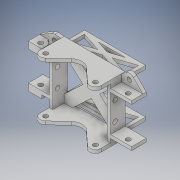
# Autodesk Inventor part: 14HM08 Chassis
Saved by Autodesk Inventor 2019 (Build 230136000, 136)
## iProperties
Created: 2019-01-31
Part Number: 14HM08 Chassis
Material: Generic
Document SubType Name: Modeling
Designer: Billy
Density: 1 g/cm^3
Appearance: Red
Author: Billy
Autodesk Inventor part; units mm, degrees
ref_plane "YZ Plane" through (0, 0, 0) normal (1, 0, 0) x (0, 1, 0)
ref_plane "XZ Plane" through (0, 0, 0) normal (0, 1, 0) x (-1, 0, 0)
ref_plane "XY Plane" through (0, 0, 0) normal (0, 0, 1) x (1, 0, 0)
sketch "Sketch1" plane through (0, 0, 0) normal (0, 1, 0) x (-1, 0, 0)
  circle A0 centre (21.95, 0) radius 2
  circle A1 centre (-21.95, 0) radius 2
  arc A2 (26.95, 0) -> (18.5331, 3.6504) centre (21.95, 0) ccw
  arc A3 (-18.5331, 3.6504) -> (-26.95, 0) centre (-21.95, 0) ccw
  arc A4 (-6.8337, -7.3007) -> (6.8337, -7.3007) centre (0, 0) ccw
  line L0 (6.8337, -7.3007) -> (18.5331, 3.6504)
  line L1 (-6.8337, -7.3007) -> (-18.5331, 3.6504)
  line L2 (-26.95, 0) -> (-26.95, -18.25)
  line L3 (-26.95, -18.25) -> (26.95, -18.25)
  line L4 (26.95, -18.25) -> (26.95, 0)
  constraints: 10 end point, 6 point on circle, 5 centre point, 4 tangent, 3 coincident, 1 parallel, 5 other
extrude "Extrusion1" add sketch "Sketch1" along normal blind 3
ref_plane "Work Plane1" through (0, 48, 0) normal (0, 1, 0) x (1, 0, 0)
sketch "Sketch2" plane through (0, 48, 0) normal (0, 1, 0) x (1, 0, 0)
  circle A0 centre (21.95, 0) radius 2 projected
  circle A1 centre (-21.95, 0) radius 2 projected
  line L0 (-18.5331, -3.6504) -> (-6.8337, 7.3007) projected
  arc A2 (6.8337, 7.3007) -> (-6.8337, 7.3007) centre (0, 0) ccw projected
  line L1 (6.8337, 7.3007) -> (18.5331, -3.6504) projected
  arc A3 (18.5331, -3.6504) -> (26.95, 0) centre (21.95, 0) ccw projected
  line L2 (26.95, 0) -> (26.95, 18.25) projected
  line L3 (26.95, 18.25) -> (-26.95, 18.25) projected
  line L4 (-26.95, 18.25) -> (-26.95, 0) projected
  arc A4 (-26.95, 0) -> (-18.5331, -3.6504) centre (-21.95, 0) ccw projected
extrude "Extrusion2" add sketch "Sketch2" along normal blind 3
sketch "Sketch3" plane through (26.95, 48, -18.25) normal (0, 0, -1) x (-1, 0, 0)
  line L0 (0, 0) -> (53.9, 0) projected
  line L1 (53.9, 0) -> (53.9, 3) projected
  line L2 (0, 3) -> (53.9, 3) projected
  line L3 (0, 0) -> (0, 3) projected
  line L4 (53.9, -48) -> (0, -48) projected
  line L5 (53.9, -48) -> (53.9, -45) projected
  line L6 (0, -45) -> (53.9, -45) projected
  line L7 (0, -48) -> (0, -45) projected
  circle A0 centre (-6.625, -46.63) radius 2
  circle A1 centre (-6.625, 1.63) radius 2
  circle A2 centre (59.415, -43.455) radius 2
  circle A3 centre (59.415, -1.545) radius 2
  arc A4 (58.9874, -48.4367) -> (59.415, -38.455) centre (59.415, -43.455) ccw
  arc A5 (-6.625, -41.63) -> (-3.6882, -50.6767) centre (-6.625, -46.63) ccw
  arc A6 (59.415, -6.545) -> (58.9874, 3.4367) centre (59.415, -1.545) ccw
  arc A7 (-3.6882, 5.6767) -> (-6.625, -3.37) centre (-6.625, 1.63) ccw
  line L8 (53.9, -48) -> (0, -48)
  line L9 (0, 3) -> (53.9, 3)
  line L10 (0, -48) -> (-3.6882, -50.6767)
  line L11 (-6.625, -41.63) -> (0, -41.63)
  line L12 (53.9, -48) -> (58.9874, -48.4367)
  line L13 (59.415, -38.455) -> (53.9, -38.455)
  line L14 (53.9, -45) -> (53.9, -48)
  line L15 (0, -48) -> (0, -45)
  line L16 (59.415, -6.545) -> (53.9, -6.545)
  line L17 (53.9, 3) -> (58.9874, 3.4367)
  line L18 (53.9, 3) -> (53.9, 0)
  line L19 (53.9, -6.545) -> (53.9, -38.455)
  line L20 (0, 3) -> (-3.6882, 5.6767)
  line L21 (-6.625, -3.37) -> (0, -3.37)
  line L22 (0, -41.63) -> (0, -3.37)
  line L23 (0, 0) -> (0, 3)
  point P0 (26.95, -48)
  constraints: 36 end point, 10 parallel, 10 perpendicular, 8 centre point, 8 point on circle, 6 tangent, 4 coincident, 2 horizontal, 2 vertical, 8 other
extrude "Extrusion3" add sketch "Sketch3" along normal blind 3
sketch "Sketch4" plane through (26.95, 0, 0) normal (1, 0, 0) x (0, 0, -1)
  line L0 (18.25, 3) -> (0, 3) projected
  line L1 (7.3007, 48) -> (10, 48) projected
  line L2 (18.25, 3) -> (8.25, 3)
  line L3 (8.25, 3) -> (8.25, 48)
  line L4 (8.25, 48) -> (18.25, 48)
  line L5 (18.25, 48) -> (18.25, 3)
  point P0 (0, 0)
  dimension "d34" = 10
  constraints: 8 end point, 2 parallel, 1 horizontal, 1 perpendicular, 1 point on line
  measures "d34" distance of L3.end L4.end
extrude "Extrusion4" add sketch "Sketch4" against normal blind 3
sketch "Sketch5" plane through (-26.95, 0, 0) normal (-1, 0, 0) x (0, 0, 1)
  line L0 (-8.25, 3) -> (-18.25, 3) projected
  line L1 (-8.25, 3) -> (-8.25, 48) projected
  line L2 (-18.25, 48) -> (-8.25, 48) projected
  line L3 (-18.25, 3) -> (-18.25, 48) projected
  point P0 (0, 0)
extrude "Extrusion5" add sketch "Sketch5" against normal blind 3
sketch "Sketch6" plane through (26.95, 48, -18.25) normal (0, 0, 1) x (1, 0, 0)
  line L0 (-50.9, -6.8604) -> (-50.9, -38.1396)
  line L1 (-10.3025, -45) -> (-43.5975, -45)
  line L2 (-3, -38.1396) -> (-3, -6.8604)
  line L3 (-10.3025, 0) -> (-43.5975, 0)
  line L4 (-50.9, -38.1396) -> (-34.2525, -22.5)
  line L5 (-26.95, -15.6396) -> (-10.3025, 0)
  line L6 (-10.3025, -45) -> (-26.95, -29.3604)
  line L7 (-34.2525, -22.5) -> (-50.9, -6.8604)
  line L8 (-3, -38.1396) -> (-19.6475, -22.5)
  line L9 (-26.95, -15.6396) -> (-43.5975, 0)
  line L10 (-43.5975, -45) -> (-26.95, -29.3604)
  line L11 (-19.6475, -22.5) -> (-3, -6.8604)
  point P0 (-26.95, -48)
  constraints: 24 end point
extrude "Extrusion6" cut sketch "Sketch6" against normal blind 3
sketch "Sketch8" plane through (26.95, 48, -21.25) normal (0, 0, -1) x (-1, 0, 0)
  line L0 (10.3025, -45) -> (26.95, -29.3604)
  line L1 (26.95, -29.3604) -> (43.5975, -45)
  line L2 (43.5975, -45) -> (10.3025, -45)
  line L3 (43.5975, 0) -> (26.95, -15.6396)
  line L4 (26.95, -15.6396) -> (10.3025, 0)
  line L5 (10.3025, 0) -> (43.5975, 0)
  line L6 (3, -6.8604) -> (19.6475, -22.5)
  line L7 (19.6475, -22.5) -> (3, -38.1396)
  line L8 (3, -38.1396) -> (3, -6.8604)
  line L9 (50.9, -38.1396) -> (34.2525, -22.5)
  line L10 (34.2525, -22.5) -> (50.9, -6.8604)
  line L11 (50.9, -6.8604) -> (50.9, -38.1396)
  circle A0 centre (59.415, -1.545) radius 2
  circle A1 centre (59.415, -43.455) radius 2
  circle A2 centre (-6.625, 1.63) radius 2
  circle A3 centre (-6.625, -46.63) radius 2
  line L12 (0, 3) -> (-3.6882, 5.6767)
  arc A4 (-3.6882, 5.6767) -> (-6.625, -3.37) centre (-6.625, 1.63) ccw
  arc A5 (-6.625, -41.63) -> (-3.6882, -50.6767) centre (-6.625, -46.63) ccw
  line L13 (-3.6882, -50.6767) -> (0, -48)
  line L14 (0, -48) -> (53.9, -48)
  line L15 (53.9, -48) -> (58.9874, -48.4367)
  arc A6 (58.9874, -48.4367) -> (59.415, -38.455) centre (59.415, -43.455) ccw
  line L16 (59.415, -38.455) -> (53.9, -38.455)
  line L17 (57.122, -6.545) -> (59.415, -6.545)
  arc A7 (59.415, -6.545) -> (58.9874, 3.4367) centre (59.415, -1.545) ccw
  line L18 (58.9874, 3.4367) -> (53.9, 3)
  line L19 (53.9, 3) -> (0, 3)
  line L20 (53.9, -40.75) -> (0, -40.75)
  line L21 (53.9, -4.25) -> (0, -4.25)
  line L22 (0, -41.63) -> (0, -43.75)
  line L23 (0, -1.25) -> (0, -4.25)
  line L24 (0, -40.75) -> (0, -41.63)
  line L25 (63.6201, -43.75) -> (57.4369, -43.75)
  line L26 (53.9, -43.75) -> (0, -43.75)
  line L27 (63.6201, -1.25) -> (57.4369, -1.25)
  line L28 (53.9, -1.25) -> (0, -1.25)
  line L29 (53.9, -43.75) -> (53.9, -40.75)
  line L30 (53.9, -4.25) -> (53.9, -1.25)
  point P0 (26.95, -48)
  constraints: 62 end point, 8 centre point, 4 point on circle, 1 point on line, 18 other
extrude "Extrusion7" add sketch "Sketch8" along normal blind 18 contours L26 L22 L24 L20 L0 | L0 L20 L1 L26 | L1 L20 L29 L26 | L28 L30 L21 L3 | L3 L21 L4 L28 | L4 L21 L23 L28
sketch "Sketch9" plane through (-12.1236, 43.75, -21.25) normal (0, -1, 0) x (1, 0, 0)
  line L0 (24.2473, 0) -> (39.0736, 0)
  line L1 (24.2473, 0) -> (0, 0)
  line L2 (-14.8264, 0) -> (0, 0)
  line L3 (-14.8264, 0) -> (-14.8264, -18)
  line L4 (39.0736, -18) -> (-14.8264, -18)
  line L5 (39.0736, 0) -> (39.0736, -18)
  line L6 (-11.8264, -15) -> (-11.8264, -3)
  line L7 (0, -3) -> (24.2473, -3)
  line L8 (36.0736, -3) -> (36.0736, -15)
  line L9 (23.7763, -15) -> (0.471, -15)
  line L10 (-8.5123, -18) -> (-14.1928, -19.897)
  line L11 (38.4401, -19.897) -> (32.7596, -18)
  line L12 (12.1236, -11.1086) -> (0.471, -15)
  line L13 (23.7763, -15) -> (12.1236, -11.1086)
  line L14 (5.8096, -9) -> (-11.8264, -14.8896)
  line L15 (-14.8264, -15.8914) -> (-15.4599, -16.103)
  line L16 (5.8096, -9) -> (-11.8264, -3.1104)
  line L17 (-14.8264, -2.1086) -> (-15.4599, -1.897)
  line L18 (38.4401, 1.897) -> (32.7596, 0)
  line L19 (23.7763, -3) -> (12.1236, -6.8914)
  line L20 (-8.5123, 0) -> (-14.1928, 1.897)
  line L21 (12.1236, -6.8914) -> (0.471, -3)
  line L22 (39.7072, -16.103) -> (39.0736, -15.8914)
  line L23 (36.0736, -14.8896) -> (18.4377, -9)
  line L24 (39.7072, -1.897) -> (39.0736, -2.1086)
  line L25 (36.0736, -3.1104) -> (18.4377, -9)
  point P0 (12.1236, 21.25)
  dimension "d62" = 3
  constraints: 52 end point, 14 point on line
  measures "d62" distance between parallel lines of L4 L9
extrude "Extrusion8" cut sketch "Sketch9" along normal blind 180 and the other way blind 9 contours L6 L16 L14 | L7 L19 L21 | L8 L23 L25 | L9 L12 L13
sketch "Sketch13" plane through (26.95, 48, -21.25) normal (0, 0, -1) x (-1, 0, 0)
  line L0 (-6.625, -3.37) -> (0, -3.37)
  line L1 (0, -3.37) -> (-6.625, -3.37)
  line L2 (-11.625, 1.63) -> (-11.625, -6.37)
  line L3 (-11.625, -6.37) -> (0, -6.37)
  line L4 (0, -6.37) -> (0, -3.37)
  line L5 (0, -1.25) -> (11.633, -1.25) projected
  line L6 (11.633, -1.25) -> (10.3025, 0) projected
  line L7 (10.3025, 0) -> (43.5975, 0) projected
  line L8 (43.5975, 0) -> (42.267, -1.25) projected
  line L9 (42.267, -1.25) -> (53.9, -1.25) projected
  line L10 (53.9, -1.25) -> (53.9, -4.25) projected
  line L11 (53.9, -4.25) -> (39.0736, -4.25) projected
  line L12 (39.0736, -4.25) -> (26.95, -15.6396) projected
  line L13 (26.95, -15.6396) -> (14.8264, -4.25) projected
  line L14 (14.8264, -4.25) -> (0, -4.25) projected
  line L15 (0, -4.25) -> (0, -40.75) projected
  line L16 (0, -40.75) -> (14.8264, -40.75) projected
  line L17 (14.8264, -40.75) -> (26.95, -29.3604) projected
  line L18 (26.95, -29.3604) -> (39.0736, -40.75) projected
  line L19 (39.0736, -40.75) -> (53.9, -40.75) projected
  line L20 (53.9, -40.75) -> (53.9, -43.75) projected
  line L21 (53.9, -43.75) -> (42.267, -43.75) projected
  line L22 (42.267, -43.75) -> (43.5975, -45) projected
  line L23 (43.5975, -45) -> (10.3025, -45) projected
  line L24 (10.3025, -45) -> (11.633, -43.75) projected
  line L25 (11.633, -43.75) -> (0, -43.75) projected
  line L26 (0, -43.75) -> (0, -43.3734)
  line L27 (0, -41.63) -> (-6.625, -41.63)
  arc A0 (-6.625, -41.63) -> (-11.625, -46.63) centre (-6.625, -46.63) ccw
  line L28 (-3.6882, -50.6767) -> (0, -48)
  line L29 (0, -48) -> (53.9, -48) projected
  line L30 (53.9, -48) -> (58.9874, -48.4367) projected
  arc A1 (58.9874, -48.4367) -> (59.415, -38.455) centre (59.415, -43.455) ccw projected
  line L31 (59.415, -38.455) -> (53.9, -38.455) projected
  line L32 (53.9, -38.455) -> (53.9, -6.545) projected
  line L33 (53.9, -6.545) -> (59.415, -6.545) projected
  arc A2 (59.415, -6.545) -> (58.9874, 3.4367) centre (59.415, -1.545) ccw projected
  line L34 (58.9874, 3.4367) -> (53.9, 3) projected
  line L35 (53.9, 3) -> (0, 3) projected
  line L36 (0, 3) -> (-3.6882, 5.6767)
  arc A3 (-11.625, 1.63) -> (-6.625, -3.37) centre (-6.625, 1.63) ccw
  line L37 (-6.625, -3.37) -> (0, -3.37)
  line L38 (0, -3.37) -> (0, -1.25)
  line L39 (3, -6.8604) -> (19.6475, -22.5) projected
  line L40 (19.6475, -22.5) -> (3, -38.1396) projected
  line L41 (3, -38.1396) -> (3, -6.8604) projected
  line L42 (50.9, -38.1396) -> (34.2525, -22.5) projected
  line L43 (34.2525, -22.5) -> (50.9, -6.8604) projected
  line L44 (50.9, -6.8604) -> (50.9, -38.1396) projected
  circle A4 centre (59.415, -1.545) radius 2 projected
  circle A5 centre (59.415, -43.455) radius 2 projected
  circle A6 centre (-6.625, 1.63) radius 2
  circle A7 centre (-6.625, -46.63) radius 2
  line L45 (0, -41.63) -> (-6.625, -41.63)
  line L46 (-11.625, -46.63) -> (-11.625, -38.63)
  line L47 (-11.625, -38.63) -> (0, -38.63)
  line L48 (0, -38.63) -> (0, -41.63)
  point P0 (26.95, -48)
  constraints: 30 end point, 12 centre point, 4 point on circle, 1 point on line
extrude "Extrusion11" add sketch "Sketch13" against normal up to surface (3 mm away) contours L0 L4 L3 L2 A3 | L15 L48 L27 A0 L46 L47
sketch "Sketch14" plane through (26.95, 48, -18.25) normal (0, 0, 1) x (1, 0, 0)
  line L0 (0, -48) -> (0, -38.63) projected
  line L1 (3.6882, -50.6767) -> (0, -48) projected
  arc A0 (3.6882, -50.6767) -> (11.625, -46.63) centre (6.625, -46.63) ccw projected
  line L2 (11.625, -38.63) -> (11.625, -46.63) projected
  line L3 (0, -38.63) -> (11.625, -38.63) projected
  circle A1 centre (6.625, -46.63) radius 2 projected
  circle A2 centre (6.625, 1.63) radius 2 projected
  line L4 (0, -6.37) -> (0, 3) projected
  line L5 (11.625, -6.37) -> (0, -6.37) projected
  line L6 (11.625, 1.63) -> (11.625, -6.37) projected
  arc A3 (11.625, 1.63) -> (3.6882, 5.6767) centre (6.625, 1.63) ccw projected
  line L7 (0, 3) -> (3.6882, 5.6767) projected
  line L8 (0, -1.25) -> (0, -4.25) projected
  line L9 (11.625, -6.37) -> (0, -6.37)
  line L10 (0, -6.37) -> (0, -3.37)
  line L11 (0, -3.37) -> (11.625, -3.37)
  line L12 (11.625, -3.37) -> (11.625, -6.37)
  line L13 (11.625, -38.63) -> (0, -38.63)
  line L14 (0, -38.63) -> (0, -41.63)
  line L15 (0, -41.63) -> (11.625, -41.63)
  line L16 (11.625, -41.63) -> (11.625, -38.63)
  point P0 (-26.95, -48)
  dimension "d92" = 3
  dimension "d93" = 3
  constraints: 16 end point, 4 parallel, 2 horizontal, 2 perpendicular, 2 point on line
  measures "d92" distance of L9.end L10.end
  measures "d93" distance of L14.end L13.end
extrude "Extrusion12" add sketch "Sketch14" along normal blind 10 contours L0 L3 L2 L15 | L4 L11 L6 L5
sketch "Sketch15" plane through (38.575, 41.63, -21.25) normal (1, 0, 0) x (0, 0, -1)
  line L0 (-3, -35.26) -> (-3, -40.26) projected
  line L1 (-3, -40.26) -> (0, -40.26) projected
  line L2 (0, -32.26) -> (0, -40.26) projected
  line L3 (0, -32.26) -> (-13, -32.26) projected
  line L4 (-13, -35.26) -> (-13, -32.26) projected
  line L5 (-3, -35.26) -> (-13, -35.26) projected
  line L6 (-3, 8) -> (-3, 3) projected
  line L7 (-3, 3) -> (-13, 3) projected
  line L8 (-13, 0) -> (-13, 3) projected
  line L9 (0, 0) -> (-13, 0) projected
  line L10 (0, 8) -> (0, 0) projected
  line L11 (-3, 8) -> (0, 8) projected
  line L12 (0, -32.26) -> (-13, -32.26) projected
  line L13 (-13, -35.26) -> (0, -35.26)
  line L14 (0, -35.26) -> (0, -32.26)
  line L15 (0, -32.26) -> (-13, -32.26)
  line L16 (-13, -32.26) -> (-13, -35.26)
  line L17 (-13, 0) -> (0, 0)
  line L18 (0, 0) -> (0, 3)
  line L19 (0, 3) -> (-13, 3)
  line L20 (-13, 3) -> (-13, 0)
  point P0 (-21.25, -41.63)
  constraints: 16 end point, 4 parallel, 2 horizontal, 2 perpendicular, 1 point on line
extrude "Extrusion13" add sketch "Sketch15" along normal blind 7 contours L5 L4 L3 L2 L13 | L19 L10 L9 L8 L7
sketch "Sketch16" plane through (26.95, 44.63, -18.25) normal (0, 1, 0) x (1, 0, 0)
  line L0 (0, 0) -> (11.625, 0) projected
  line L1 (0, -10) -> (0, 0) projected
  line L2 (0, -10) -> (18.625, -10) projected
  line L3 (18.625, 3) -> (18.625, -10) projected
  line L4 (11.625, 3) -> (18.625, 3) projected
  line L5 (11.625, 0) -> (11.625, 3) projected
  line L6 (18.625, -10) -> (11.625, -10)
  line L7 (11.625, -6) -> (18.625, -6)
  line L8 (18.625, -6) -> (18.625, -10)
  circle A0 centre (11.625, -6) radius 2
  point P0 (-26.95, -18.25)
  dimension "d98" = 7
  dimension "d99" = 4
  dimension "d100" = 4
  constraints: 6 end point, 1 centre point, 1 coincident, 1 horizontal, 1 parallel
  measures "d98" distance of L7.start L7.end
  measures "d99" distance of L6.end L7.start
  measures "d100" diameter of A0
extrude "Extrusion14" cut sketch "Sketch16" along normal blind 100 and the other way blind 200 contours A0
sketch "Sketch17" plane through (26.95, 48, -18.25) normal (0, 0, 1) x (1, 0, 0)
  circle A0 centre (-59.415, -1.545) radius 2
  line L0 (-58.9874, 3.4367) -> (-53.9, 3)
  arc A1 (-64.4104, -1.759) -> (-59.415, -6.545) centre (-59.415, -1.545) ccw
  line L1 (-53.9, -6.545) -> (-59.415, -6.545)
  line L2 (-59.415, -38.455) -> (-53.9, -38.455)
  arc A2 (-59.415, -38.455) -> (-64.4104, -43.241) centre (-59.415, -43.455) ccw
  line L3 (-53.9, -48) -> (-58.9874, -48.4367)
  circle A3 centre (-59.415, -43.455) radius 2
  line L4 (-53.9, -6.545) -> (-59.415, -6.545)
  line L5 (-64.4104, -1.759) -> (-64.4104, -9.545)
  line L6 (-64.4104, -9.545) -> (-53.9, -9.545)
  line L7 (-53.9, -9.545) -> (-53.9, -6.545)
  line L8 (-53.9, -38.455) -> (-59.415, -38.455)
  line L9 (-64.4104, -43.241) -> (-64.4104, -35.455)
  line L10 (-64.4104, -35.455) -> (-53.9, -35.455)
  line L11 (-53.9, -35.455) -> (-53.9, -38.455)
  point P0 (-26.95, -48)
  constraints: 24 end point, 8 centre point, 4 point on circle
extrude "Extrusion15" add sketch "Sketch17" against normal up to surface (3 mm away) contours A1 L1 L7 L6 L5 | A2 L9 L10 L11 L2
sketch "Sketch19" plane through (26.95, 48, -18.25) normal (0, 0, 1) x (1, 0, 0)
  circle A0 centre (-59.415, -1.545) radius 2 projected
  line L0 (-53.9, 3) -> (-53.9, -9.545) projected
  line L1 (-58.9874, 3.4367) -> (-53.9, 3) projected
  arc A1 (-58.9874, 3.4367) -> (-64.4104, -1.759) centre (-59.415, -1.545) ccw projected
  line L2 (-64.4104, -1.759) -> (-64.4104, -9.545) projected
  line L3 (-64.4104, -9.545) -> (-53.9, -9.545) projected
  line L4 (-53.9, -35.455) -> (-53.9, -48) projected
  line L5 (-53.9, -35.455) -> (-64.4104, -35.455) projected
  line L6 (-64.4104, -35.455) -> (-64.4104, -43.241) projected
  arc A2 (-64.4104, -43.241) -> (-58.9874, -48.4367) centre (-59.415, -43.455) ccw projected
  line L7 (-53.9, -48) -> (-58.9874, -48.4367) projected
  circle A3 centre (-59.415, -43.455) radius 2 projected
  line L8 (-64.4104, -9.545) -> (-53.9, -9.545) projected
  line L9 (-64.4104, -9.545) -> (-53.9, -9.545)
  line L10 (-53.9, -9.545) -> (-53.9, -6.545)
  line L11 (-53.9, -6.545) -> (-64.4104, -6.545)
  line L12 (-64.4104, -6.545) -> (-64.4104, -9.545)
  line L13 (-53.9, -45) -> (-53.9, 0) projected
  line L14 (-64.4104, -35.455) -> (-53.9, -35.455)
  line L15 (-53.9, -35.455) -> (-53.9, -38.455)
  line L16 (-53.9, -38.455) -> (-64.4104, -38.455)
  line L17 (-64.4104, -38.455) -> (-64.4104, -35.455)
  point P0 (-26.95, -48)
  dimension "d110" = 3
  dimension "d111" = 3
  constraints: 16 end point, 4 parallel, 2 horizontal, 2 perpendicular, 2 point on line
  measures "d110" distance of L10.end L9.end
  measures "d111" distance of L14.end L15.end
extrude "Extrusion16" add sketch "Sketch19" along normal up to surface (10 mm away) contours L0 L3 L2 L11 | L4 L16 L6 L5
sketch "Sketch20" plane through (-37.4604, 38.455, -21.25) normal (-1, 0, 0) x (0, 0, 1)
  line L0 (0, 7.786) -> (0, 0) projected
  line L1 (0, 0) -> (13, 0) projected
  line L2 (13, 0) -> (13, 3) projected
  line L3 (3, 3) -> (13, 3) projected
  line L4 (3, 7.786) -> (3, 3) projected
  line L5 (0, 7.786) -> (3, 7.786) projected
  line L6 (0, -25.91) -> (0, -33.696) projected
  line L7 (3, -33.696) -> (0, -33.696) projected
  line L8 (3, -28.91) -> (3, -33.696) projected
  line L9 (3, -28.91) -> (13, -28.91) projected
  line L10 (13, -28.91) -> (13, -25.91) projected
  line L11 (0, -25.91) -> (13, -25.91) projected
  line L12 (13, 3) -> (0, 3)
  line L13 (0, 3) -> (0, 0)
  line L14 (0, 0) -> (13, 0)
  line L15 (13, 0) -> (13, 3)
  line L16 (13, -28.91) -> (13, -25.91) projected
  line L17 (0, -25.91) -> (13, -25.91)
  line L18 (13, -25.91) -> (13, -28.91)
  line L19 (13, -28.91) -> (0, -28.91)
  line L20 (0, -28.91) -> (0, -25.91)
  point P0 (21.25, -38.455)
  constraints: 16 end point, 4 parallel, 2 horizontal, 2 perpendicular
extrude "Extrusion17" add sketch "Sketch20" along normal blind 8.115 contours L12 L3 L2 L1 L0 | L11 L10 L9 L19 L6
sketch "Sketch21" plane through (-37.4604, 41.455, -18.25) normal (0, 1, 0) x (1, 0, 0)
  line L0 (10.5104, -10) -> (-8.115, -10) projected
  line L1 (-8.115, -10) -> (-1.115, -10)
  line L2 (-1.115, -6) -> (-8.115, -6)
  line L3 (-8.115, -6) -> (-8.115, -10)
  circle A0 centre (-1.115, -6) radius 2
  point P0 (37.4604, -18.25)
  dimension "d116" = 7
  dimension "d117" = 4
  dimension "d118" = 4
  constraints: 6 end point, 1 centre point, 1 coincident, 1 horizontal, 1 parallel
  measures "d116" distance of L2.end L2.start
  measures "d117" distance of L2.start L1.end
  measures "d118" diameter of A0
extrude "Extrusion18" cut sketch "Sketch21" against normal blind 50.49
sketch "Sketch22" plane through (-37.4604, 41.455, -18.25) normal (0, 1, 0) x (1, 0, 0)
  circle A0 centre (-1.115, -6) radius 2 projected
  arc A1 (3.885, -6) -> (0, -1.1259) centre (-1.115, -6) ccw
  circle A2 centre (-1.115, -6) radius 2 projected
  line L0 (10.5104, -10) -> (-8.115, -10) projected
  line L1 (10.5104, 0) -> (10.5104, -10) projected
  line L2 (0, 0) -> (10.5104, 0) projected
  line L3 (0, 3) -> (0, 0) projected
  line L4 (0, 3) -> (-8.115, 3) projected
  line L5 (-8.115, -10) -> (-8.115, 3) projected
  line L6 (3.885, -6) -> (3.885, -10)
  line L7 (0, 0) -> (0, -1.1259)
  point P0 (37.4604, -18.25)
  dimension "d121" = 10
  constraints: 4 end point, 2 point on circle, 2 vertical, 1 centre point, 1 coincident, 1 point on line
  measures "d121" diameter of A1
extrude "Extrusion19" add sketch "Sketch22" along normal blind 3.175 contours L6 L0 L5 L4 L3 L7 A1
sketch "Sketch23" plane through (-37.4604, 9.545, -18.25) normal (0, -1, 0) x (1, 0, 0)
  circle A0 centre (-1.115, 6) radius 2 projected
  line L0 (-8.115, 10) -> (3.885, 10) projected
  line L1 (3.885, 10) -> (3.885, 6) projected
  arc A1 (0, 1.1259) -> (3.885, 6) centre (-1.115, 6) ccw projected
  line L2 (0, 1.1259) -> (0, 0) projected
  line L3 (0, -3) -> (0, 0) projected
  line L4 (0, -3) -> (-8.115, -3) projected
  line L5 (-8.115, -3) -> (-8.115, 10) projected
  point P0 (37.4604, 18.25)
extrude "Extrusion20" add sketch "Sketch23" along normal blind 3.175
sketch "Sketch24" plane through (26.95, 48, -21.25) normal (0, 0, -1) x (-1, 0, 0)
  line L0 (0, -6.37) -> (0, -38.63)
  line L1 (0, -38.63) -> (-18.625, -38.63)
  line L2 (-18.625, -41.63) -> (-18.625, -38.63)
  line L3 (-11.625, -41.63) -> (-18.625, -41.63)
  line L4 (-11.625, -41.63) -> (-11.625, -46.63)
  arc A0 (-11.625, -46.63) -> (-3.6882, -50.6767) centre (-6.625, -46.63) ccw
  line L5 (-3.6882, -50.6767) -> (0, -48)
  line L6 (0, -48) -> (53.9, -48)
  line L7 (53.9, -48) -> (58.9874, -48.4367)
  arc A1 (58.9874, -48.4367) -> (64.4104, -43.241) centre (59.415, -43.455) ccw
  line L8 (64.4104, -40.955) -> (64.4104, -43.241)
  line L9 (72.5254, -40.955) -> (64.4104, -40.955)
  line L10 (72.5254, -35.455) -> (72.5254, -40.955)
  line L11 (53.9, -35.455) -> (72.5254, -35.455)
  line L12 (53.9, -35.455) -> (53.9, -9.545)
  line L13 (53.9, -9.545) -> (72.5254, -9.545)
  line L14 (72.5254, -9.545) -> (72.5254, -4.045)
  line L15 (64.4104, -4.045) -> (72.5254, -4.045)
  line L16 (64.4104, -1.759) -> (64.4104, -4.045)
  arc A2 (64.4104, -1.759) -> (58.9874, 3.4367) centre (59.415, -1.545) ccw
  line L17 (58.9874, 3.4367) -> (53.9, 3)
  line L18 (53.9, 3) -> (0, 3)
  line L19 (0, 3) -> (-3.6882, 5.6767)
  arc A3 (-3.6882, 5.6767) -> (-11.625, 1.63) centre (-6.625, 1.63) ccw
  line L20 (-11.625, 1.63) -> (-11.625, -3.37)
  line L21 (-11.625, -3.37) -> (-18.625, -3.37)
  line L22 (-18.625, -6.37) -> (-18.625, -3.37)
  line L23 (-18.625, -6.37) -> (0, -6.37)
  line L24 (0, -1.25) -> (0, -4.25)
  line L25 (0, -1.25) -> (11.633, -1.25)
  line L26 (11.633, -1.25) -> (10.3025, 0)
  line L27 (10.3025, 0) -> (43.5975, 0)
  line L28 (43.5975, 0) -> (42.267, -1.25)
  line L29 (42.267, -1.25) -> (53.9, -1.25)
  line L30 (53.9, -1.25) -> (53.9, -4.25)
  line L31 (53.9, -4.25) -> (39.0736, -4.25)
  line L32 (39.0736, -4.25) -> (26.95, -15.6396)
  line L33 (26.95, -15.6396) -> (14.8264, -4.25)
  line L34 (14.8264, -4.25) -> (0, -4.25)
  line L35 (0, -40.75) -> (0, -43.75)
  line L36 (0, -40.75) -> (14.8264, -40.75)
  line L37 (14.8264, -40.75) -> (26.95, -29.3604)
  line L38 (26.95, -29.3604) -> (39.0736, -40.75)
  line L39 (39.0736, -40.75) -> (53.9, -40.75)
  line L40 (53.9, -40.75) -> (53.9, -43.75)
  line L41 (53.9, -43.75) -> (42.267, -43.75)
  line L42 (42.267, -43.75) -> (43.5975, -45)
  line L43 (43.5975, -45) -> (10.3025, -45)
  line L44 (10.3025, -45) -> (11.633, -43.75)
  line L45 (11.633, -43.75) -> (0, -43.75)
  line L46 (3, -6.8604) -> (19.6475, -22.5)
  line L47 (19.6475, -22.5) -> (3, -38.1396)
  line L48 (3, -38.1396) -> (3, -6.8604)
  line L49 (50.9, -38.1396) -> (34.2525, -22.5)
  line L50 (34.2525, -22.5) -> (50.9, -6.8604)
  line L51 (50.9, -6.8604) -> (50.9, -38.1396)
  circle A4 centre (59.415, -1.545) radius 2
  circle A5 centre (59.415, -43.455) radius 2
  circle A6 centre (-6.625, 1.63) radius 2
  circle A7 centre (-6.625, -46.63) radius 2
  line L52 (-18.625, -3.37) -> (-10.1753, 5.1507)
  arc A8 (-3.6882, 5.6767) -> (-11.625, 1.63) centre (-6.625, 1.63) ccw projected
  line L53 (-18.625, -41.63) -> (-10.1753, -50.1507)
  line L54 (72.5254, -4.045) -> (62.1233, 2.658)
  line L55 (72.5254, -40.955) -> (62.1233, -47.658)
  point P0 (26.95, -48)
  point P1 (64.4104, -2.902)
  constraints: 112 end point, 16 centre point, 12 point on circle, 6 vertical, 4 horizontal, 4 tangent, 1 midpoint, 6 other
extrude "Extrusion21" add sketch "Sketch24" against normal up to surface (3 mm away) contours L52 A3 L20 L21 | L3 L4 A0 L53 | L54 L15 L16 A2 | A1 L8 L9 L55
sketch "Sketch25" plane through (26.95, 9.37, -8.25) normal (1, 0, 0) x (0, 0, -1)
  line L0 (0, 0) -> (13, 0) projected
  line L1 (13, 32.26) -> (13, 0) projected
  line L2 (13, 32.26) -> (0, 32.26) projected
  line L3 (0, 0) -> (0, 32.26) projected
  line L4 (13, 32.26) -> (0, 32.26) projected
  line L5 (0, 32.26) -> (4, 32.26)
  line L6 (4, 32.26) -> (4, 24.26)
  line L7 (4, 24.26) -> (0, 24.26)
  line L8 (0, 24.26) -> (0, 32.26)
  line L9 (0, 0) -> (4, 0)
  line L10 (4, 0) -> (4, 8)
  line L11 (4, 8) -> (0, 8)
  line L12 (0, 8) -> (0, 0)
  circle A0 centre (4, 24.26) radius 2
  circle A1 centre (4, 8) radius 2
  point P0 (-8.25, -9.37)
  dimension "d128" = 4
  dimension "d129" = 8
  dimension "d130" = 4
  dimension "d131" = 8
  dimension "d132" = 4
  dimension "d133" = 4
  constraints: 16 end point, 4 parallel, 2 centre point, 2 coincident, 2 horizontal, 2 perpendicular
  measures "d128" distance of L6.end L7.end
  measures "d129" distance of L5.end L6.end
  measures "d130" distance of L11.end L10.end
  measures "d131" distance of L10.end L9.end
  measures "d132" diameter of A0
  measures "d133" diameter of A1
extrude "Extrusion22" cut sketch "Sketch25" against normal blind 4 contours A1 L11 L10 | L10 L11 A1 | A0 L6 L7 | L7 L6 A0
sketch "Sketch27" plane through (-26.95, 12.545, -8.25) normal (-1, 0, 0) x (0, 0, 1)
  circle A0 centre (-4, 4.825) radius 2 projected
  circle A1 centre (-4, 21.085) radius 2 projected
  line L0 (0, -9.545) -> (-10, -9.545) projected
  line L1 (0, -9.545) -> (0, 35.455) projected
  line L2 (-10, 35.455) -> (0, 35.455) projected
  line L3 (-10, 28.5946) -> (-10, 35.455) projected
  line L4 (-10, 28.5946) -> (-13, 28.5946) projected
  line L5 (-13, -2.6846) -> (-13, 28.5946) projected
  line L6 (-10, -2.6846) -> (-13, -2.6846) projected
  line L7 (-10, -9.545) -> (-10, -2.6846) projected
  point P0 (8.25, -12.545)
extrude "Extrusion23" cut sketch "Sketch27" against normal blind 4 contours A0 | A1
sketch "Sketch28" plane through (26.95, 48, -21.25) normal (0, 0, -1) x (-1, 0, 0)
  line L0 (0, -1.25) -> (0, -4.25)
  line L1 (0, -1.25) -> (11.633, -1.25)
  line L2 (11.633, -1.25) -> (10.3025, 0)
  line L3 (10.3025, 0) -> (43.5975, 0)
  line L4 (43.5975, 0) -> (42.267, -1.25)
  line L5 (42.267, -1.25) -> (53.9, -1.25)
  line L6 (53.9, -1.25) -> (53.9, -4.25)
  line L7 (53.9, -4.25) -> (39.0736, -4.25)
  line L8 (39.0736, -4.25) -> (26.95, -15.6396)
  line L9 (26.95, -15.6396) -> (14.8264, -4.25)
  line L10 (14.8264, -4.25) -> (0, -4.25)
  line L11 (0, -40.75) -> (0, -43.75)
  line L12 (0, -40.75) -> (14.8264, -40.75)
  line L13 (14.8264, -40.75) -> (26.95, -29.3604)
  line L14 (26.95, -29.3604) -> (39.0736, -40.75)
  line L15 (39.0736, -40.75) -> (53.9, -40.75)
  line L16 (53.9, -40.75) -> (53.9, -43.75)
  line L17 (53.9, -43.75) -> (42.267, -43.75)
  line L18 (42.267, -43.75) -> (43.5975, -45)
  line L19 (43.5975, -45) -> (10.3025, -45)
  line L20 (10.3025, -45) -> (11.633, -43.75)
  line L21 (11.633, -43.75) -> (0, -43.75)
  line L22 (3, -6.8604) -> (19.6475, -22.5)
  line L23 (19.6475, -22.5) -> (3, -38.1396)
  line L24 (3, -38.1396) -> (3, -6.8604)
  line L25 (50.9, -38.1396) -> (34.2525, -22.5)
  line L26 (34.2525, -22.5) -> (50.9, -6.8604)
  line L27 (50.9, -6.8604) -> (50.9, -38.1396)
  circle A0 centre (59.415, -1.545) radius 2
  circle A1 centre (59.415, -43.455) radius 2
  circle A2 centre (-6.625, 1.63) radius 2
  circle A3 centre (-6.625, -46.63) radius 2
  line L28 (72.5254, -9.545) -> (72.5254, -3.37)
  line L29 (71.4779, -3.37) -> (72.5254, -3.37)
  line L30 (71.4779, -3.37) -> (62.1233, 2.658)
  arc A4 (62.1233, 2.658) -> (58.9874, 3.4367) centre (59.415, -1.545) ccw
  line L31 (58.9874, 3.4367) -> (53.9, 3)
  line L32 (53.9, 3) -> (0, 3)
  line L33 (0, 3) -> (-3.6882, 5.6767)
  arc A5 (-3.6882, 5.6767) -> (-10.1753, 5.1507) centre (-6.625, 1.63) ccw
  line L34 (-10.1753, 5.1507) -> (-18.625, -3.37)
  line L35 (-18.625, -6.37) -> (-18.625, -3.37)
  line L36 (-18.625, -6.37) -> (0, -6.37)
  line L37 (0, -6.37) -> (0, -38.63)
  line L38 (0, -38.63) -> (-18.625, -38.63)
  line L39 (-18.625, -41.63) -> (-18.625, -38.63)
  line L40 (-18.625, -41.63) -> (-10.1753, -50.1507)
  arc A6 (-10.1753, -50.1507) -> (-3.6882, -50.6767) centre (-6.625, -46.63) ccw
  line L41 (-3.6882, -50.6767) -> (0, -48)
  line L42 (0, -48) -> (53.9, -48)
  line L43 (53.9, -48) -> (58.9874, -48.4367)
  arc A7 (58.9874, -48.4367) -> (62.1233, -47.658) centre (59.415, -43.455) ccw
  line L44 (62.1233, -47.658) -> (71.4779, -41.63)
  line L45 (72.5254, -41.63) -> (71.4779, -41.63)
  line L46 (72.5254, -35.455) -> (72.5254, -41.63)
  line L47 (53.9, -35.455) -> (72.5254, -35.455)
  line L48 (53.9, -35.455) -> (53.9, -9.545)
  line L49 (53.9, -9.545) -> (72.5254, -9.545)
  line L50 (72.5254, -41.63) -> (61.9239, -47.78)
  line L51 (72.5254, -3.37) -> (61.9239, 2.78)
  arc A8 (58.9874, -48.4367) -> (62.1233, -47.658) centre (59.415, -43.455) ccw projected
  point P0 (26.95, -48)
  point P1 (64.4104, -38.455)
  point P2 (72.0017, -3.37)
  constraints: 104 end point, 16 centre point, 10 point on circle, 2 tangent, 2 vertical, 1 horizontal, 1 midpoint, 5 other
extrude "Extrusion24" add sketch "Sketch28" against normal up to surface (3 mm away) contours L29 L30 A4 L51 | L50 A7 L44 L45
body "Solid1"
